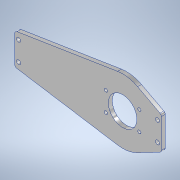
# Autodesk Inventor part: エアシリンダ側板
Saved by Autodesk Inventor 2021 (Build 250183000, 183)
## iProperties
Created: 2022-02-01
Part Number: エアシリンダ側板
Material: アルミニウム 6061
Document SubType Name: Modeling
Designer: hirohumi
Density: 2.7 g/cm^3
Appearance: アルミニウム - フラット
Mass: 43.0032 g
Surface Area: 120.025 cm^2
Volume: 15.9271 cm^3
Author: hirohumi
Autodesk Inventor part; units mm, degrees
ref_plane "YZ Plane" through (0, 0, 0) normal (1, 0, 0) x (0, 1, 0)
ref_plane "XZ Plane" through (0, 0, 0) normal (0, 1, 0) x (-1, 0, 0)
ref_plane "XY Plane" through (0, 0, 0) normal (0, 0, 1) x (1, 0, 0)
sketch "スケッチ1" plane through (0, 0, 0) normal (0, 0, 1) x (1, 0, 0)
  circle A0 centre (0, 7.5) radius 1.6
  circle A1 centre (0, -7.5) radius 1.6
  arc A2 (76.5893, 24.6922) -> (76.5893, -24.6922) centre (80.5, 0) ccw construction
  line L0 (3, 19.5) -> (75.5, 19.5) construction
  line L1 (75.5, 19.5) -> (75.5, -19.5) construction
  line L2 (75.5, -19.5) -> (3, -19.5) construction
  line L3 (3, -19.5) -> (3, 19.5) construction
  circle A3 centre (107.5, 7.5) radius 1.6
  circle A4 centre (107.5, -7.5) radius 1.6
  circle A5 centre (67.5096, 7.5) radius 1.25
  circle A6 centre (93.4904, 7.5) radius 1.25
  circle A7 centre (67.5096, -7.5) radius 1.25
  circle A8 centre (93.4904, -7.5) radius 1.25
  circle A9 centre (80.5, 0) radius 15 construction
  circle A10 centre (80.5, 0) radius 11.05
  line L4 (110.5, -12.5) -> (110.5, 12.5)
  line L5 (-3, 12.0872) -> (-3, -12.0872)
  line L6 (-3, -12.0872) -> (76.5893, -24.6922)
  line L7 (-3, 12.0872) -> (76.5893, 24.6922)
  arc A11 (80.5, 25) -> (76.5893, 24.6922) centre (80.5, 0) ccw
  arc A12 (76.5893, -24.6922) -> (80.5, -25) centre (80.5, 0) ccw
  arc A13 (80.5, -25) -> (92.1075, -22.1419) centre (80.5, 0) ccw
  line L8 (92.1075, 22.1419) -> (110.5, 12.5)
  line L9 (110.5, -12.5) -> (92.1075, -22.1419)
  arc A14 (92.1075, 22.1419) -> (80.5, 25) centre (80.5, 0) ccw
  arc A15 (92.1075, -22.1419) -> (92.1075, 22.1419) centre (80.5, 0) ccw construction
  point P0 (0, 0)
  dimension "d0" = 3.2
  dimension "d1" = 3.2
  dimension "d2" = 15
  dimension "d3" = 7.5
  dimension "d4" = 50
  dimension "d5" = 3
  dimension "d6" = 72.5
  dimension "d7" = 3.2
  dimension "d8" = 3.2
  dimension "d9" = 15
  dimension "d11" = 2.5
  dimension "d12" = 2.5
  dimension "d13" = 2.5
  dimension "d14" = 2.5
  dimension "d15" = 30
  dimension "d16" = 22.1
  dimension "d26" = 3
  dimension "d27" = 3
  dimension "d28" = 39
  dimension "d29" = 19.5
  dimension "d30" = 15
  dimension "d31" = 5
  dimension "d32" = 30
  dimension "d33" = 25
  dimension "d34" = 12.5
  dimension "d35" = 3
  dimension "d36" = 5
  dimension "d37" = 5
  constraints: 20 end point, 18 point on circle, 16 centre point, 11 tangent, 5 vertical alignment, 4 horizontal alignment, 2 coincident, 2 parallel, 1 horizontal, 1 perpendicular, 1 vertical
  measures "d0" diameter of A0
  measures "d1" diameter of A1
  measures "d2" distance of A1.centre A0.centre
  measures "d3" distance of point (0, 0) A0.centre
  measures "d4" diameter of A2
  measures "d5" distance from line of L3 A0.centre
  measures "d6" distance between parallel lines of L1 L3
  measures "d7" diameter of A3
  measures "d8" diameter of A4
  measures "d9" distance of A4.centre A3.centre
  measures "d11" diameter of A5
  measures "d12" diameter of A6
  measures "d13" diameter of A7
  measures "d14" diameter of A8
  measures "d15" diameter of A9
  measures "d16" diameter of A10
  measures "d26" distance from line of A3.centre L4
  measures "d27" distance from line of A4.centre L4
  measures "d28" distance between parallel lines of L2 L0
  measures "d29" distance from line of point (0, 0) L0
  measures "d30" distance of A7.centre A5.centre
  measures "d31" distance from line of L1 A9.centre
  measures "d32" distance from line of A2.centre L4
  measures "d33" distance of L4.start L4.end
  measures "d34" vertical distance of A2.centre L4.end
  measures "d35" distance from line of A1.centre L5
  measures "d36" distance from line of A0.centre L7
  measures "d37" distance from line of L6 A1.centre
extrude "押し出し2" add sketch "スケッチ1" along normal blind 3
fillet "フィレット2" radius 2 4 edges at (-3, 12.0872, 1.5) (-3, -12.0872, 1.5) (110.5, 12.5, 1.5) (110.5, -12.5, 1.5)
equation "\"d3\" = 0.5 * d2"
